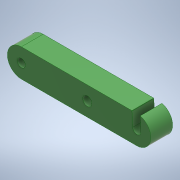
# Autodesk Inventor part: 071_0100_Base
Saved by Autodesk Inventor 2020 (Build 240168000, 168)
## iProperties
Created: 2018-07-06
Part Number: 071_0100_Base
Material: Generic
Document SubType Name: Modeling
Designer: deniz
Density: 1 g/cm^3
Appearance: Default
Author: deniz
Autodesk Inventor part; units mm, degrees
ref_plane "YZ Plane" through (0, 0, 0) normal (1, 0, 0) x (0, 1, 0)
ref_plane "XZ Plane" through (0, 0, 0) normal (0, 1, 0) x (-1, 0, 0)
ref_plane "XY Plane" through (0, 0, 0) normal (0, 0, 1) x (1, 0, 0)
sketch "Sketch1" plane through (0, 0, 0) normal (0, 1, 0) x (-1, 0, 0)
  line L0 (0, 0) -> (-74.246, 0) construction
  line L1 (0, -9) -> (-74.246, -9)
  line L2 (-74.246, 9) -> (0, 9)
  arc A0 (0, -9) -> (0, 9) centre (0, 0) ccw
  arc A1 (-74.246, 9) -> (-74.246, -9) centre (-74.246, 0) ccw
  circle A2 centre (0, 0) radius 2.6
  arc A3 (-73.6985, 9) -> (-74.246, 0) centre (0, 0) ccw construction
  arc A4 (-76.329, 9.3212) -> (-76.896, 0) centre (0, 0) ccw
  arc A5 (-71.068, 8.6788) -> (-71.596, 0) centre (0, 0) ccw
  arc A6 (-71.068, 8.6788) -> (-76.329, 9.3212) centre (-73.6985, 9) ccw
  arc A7 (-76.896, 0) -> (-71.596, 0) centre (-74.246, 0) ccw
  circle A8 centre (-42.426, 0) radius 2.95
  circle A9 centre (-42.426, 0) radius 6
  point P0 (-37.123, 0)
  dimension "d8" = 74.246
  dimension "d9" = 5.2
  dimension "d10" = 18
  dimension "d11" = 5.3
  dimension "d12" = 5.9
  dimension "d13" = 42.426
  dimension "d18" = 12
  constraints: 14 point on circle, 10 centre point, 8 end point, 8 tangent, 3 coincident, 2 point on line, 1 horizontal, 1 midpoint, 1 parallel
  measures "d8" distance of L0.start L0.end
  measures "d9" diameter of A2
  measures "d10" distance between parallel lines of L1 L2
  measures "d11" diameter of A6
  measures "d12" diameter of A8
  measures "d13" distance of L0.start A8.centre
  measures "d18" diameter of A9
extrude "Extrusion3" add sketch "Sketch1" along normal blind 4 contours L1 A1 A4 A7 A5 A6 L2 A0 | A1 L2 A6 A5 A7 A4 | A9
extrude "Extrusion4" cut sketch "Sketch1" along normal blind 10 contours A4 A6 L2 A1 | A1 L2 A6 A5 A7 A4
extrude "Extrusion5" [suppressed]
move faces "Move1" translate (0, -10, 0) faces at (38.7721, 0, -6.9762)
body "Solid2"
